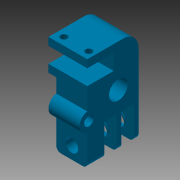
# Autodesk Inventor part: Part3
Saved by Autodesk Inventor 2015 (Build 190159000, 159)
## iProperties
Created: 2015-07-07
Part Number: Part3
Material: ABS Plastic
Document SubType Name: Modeling
Designer: eefred
Density: 1.06 g/cm^3
Appearance: Sky Blue Medium
Author: eefred
Autodesk Inventor part; units mm, degrees
ref_plane "YZ Plane" through (0, 0, 0) normal (1, 0, 0) x (0, 1, 0)
ref_plane "XZ Plane" through (0, 0, 0) normal (0, 1, 0) x (-1, 0, 0)
ref_plane "XY Plane" through (0, 0, 0) normal (0, 0, 1) x (1, 0, 0)
sketch "Sketch1" plane through (0, 0, 0) normal (1, 0, 0) x (0, 1, 0)
  line L0 (0, 0) -> (0, -5)
  line L1 (0, -5) -> (17, -5)
  line L2 (17, -5) -> (17, -15)
  line L3 (17, -15) -> (0, -15)
  line L4 (0, -61) -> (33, -61)
  line L5 (33, -61) -> (33, 0)
  line L6 (33, 0) -> (0, 0)
  circle A0 centre (1, -35) radius 3
  arc A1 (0, -29.0839) -> (0, -40.9161) centre (1, -35) ccw
  line L7 (0, -15) -> (0, -29.0839)
  line L8 (0, -61) -> (0, -40.9161)
  dimension "d0" = 5
  dimension "d1" = 17
  dimension "d2" = 10
  dimension "d4" = 33
  dimension "d6" = 6
  dimension "d7" = 1
  dimension "d8" = 20
  dimension "d9" = 6
  dimension "d47" = 46
  constraints: 18 end point, 5 perpendicular, 3 vertical, 2 centre point, 2 point on circle, 2 point on line, 1 coincident, 1 horizontal
  measures "d0" distance of L0.start L0.end
  measures "d1" distance of L0.end L1.end
  measures "d2" distance of L1.end L2.end
  measures "d4" distance of L4.start L4.end
  measures "d6" diameter of A0
  measures "d7" horizontal distance of L0.start A0.centre
  measures "d8" distance from line of L3 A0.centre
  measures "d9" radius of A1
  measures "d47" distance between parallel lines of L4 L3
extrude "Extrusion1" add sketch "Sketch1" along normal blind 25
sketch "Sketch2" plane through (0, 0, 0) normal (-1, 0, 0) x (0, 0, 1)
  line L0 (-70, -8) -> (-20, -8)
  line L1 (-20, -8) -> (-20, 42)
  line L2 (-20, 42) -> (-70, 42)
  line L3 (-70, 42) -> (-70, -8)
  point P0 (0, 0)
  dimension "d12" = 20
  dimension "d13" = 8
  dimension "d14" = 50
  dimension "d15" = 50
  constraints: 8 end point, 2 parallel, 1 horizontal, 1 perpendicular
  measures "d12" distance from line of point (0, 0) L1
  measures "d13" distance from line of point (0, 0) L0
  measures "d14" distance of L0.start L0.end
  measures "d15" distance of L2.end L0.start
extrude "Extrusion2" cut sketch "Sketch2" against normal blind 5
sketch "Sketch3" plane through (5, 0, 0) normal (-1, 0, 0) x (0, 0, 1)
  line L0 (-61, 22) -> (-40, 22)
  line L1 (-40, 22) -> (-40, 30)
  line L2 (-40, 30) -> (-61, 30)
  line L3 (-61, 30) -> (-61, 22)
  line L4 (-61, 11) -> (-40, 11)
  line L5 (-40, 11) -> (-40, 19)
  line L6 (-40, 19) -> (-61, 19)
  line L7 (-61, 19) -> (-61, 11)
  line L8 (-61, 33) -> (-20, 33) projected
  point P0 (0, 0)
  dimension "d18" = 8
  dimension "d19" = 8
  dimension "d20" = 21
  dimension "d21" = 3
  dimension "d22" = 3
  constraints: 16 end point, 4 parallel, 2 horizontal, 2 perpendicular, 2 point on line, 1 vertical alignment
  measures "d18" distance of L6.end L4.start
  measures "d19" distance of L2.end L0.start
  measures "d20" distance of L1.end L2.end
  measures "d21" distance between parallel lines of L0 L6
  measures "d22" distance between parallel lines of L8 L2
extrude "Extrusion3" cut sketch "Sketch3" against normal up to next
sketch "Sketch4" plane through (0, 33, 0) normal (0, 1, 0) x (1, 0, 0)
  circle A0 centre (15, 53) radius 4.1
  line L0 (5, 61) -> (25, 61) projected
  point P0 (0, 0)
  point P1 (15, 61)
  dimension "d25" = 8.2
  dimension "d26" = 8
  constraints: 1 centre point, 1 midpoint, 1 vertical alignment
  measures "d25" diameter of A0
  measures "d26" distance from line of L0 A0.centre
extrude "Extrusion4" cut sketch "Sketch4" against normal through all
sketch "Sketch5" plane through (5, 11, -40) normal (0, 1, 0) x (1, 0, 0)
  circle A0 centre (10, 13) radius 4.1 projected
  circle A1 centre (10, 13) radius 5
  point P0 (-5, -40)
  dimension "d29" = 10
  constraints: 1 centre point, 1 coincident
  measures "d29" diameter of A1
extrude "Extrusion5" add sketch "Sketch5" along normal blind 0.5
pattern_linear "Rectangular Pattern1" count 2 spacing 11 along (0, 1, 0) of "Extrusion5"
pattern_linear "Rectangular Pattern2" count 2 spacing 7.5 along (0, 1, 0) of "Extrusion5", "Rectangular Pattern1"
sketch "Sketch6" plane through (25, 0, 0) normal (1, 0, 0) x (0, 0, -1)
  circle A0 centre (27, 20) radius 6
  line L0 (61, 33) -> (0, 33) projected
  line L1 (0, 33) -> (0, 0) projected
  dimension "d38" = 12
  dimension "d39" = 13
  dimension "d40" = 27
  constraints: 1 centre point
  measures "d38" diameter of A0
  measures "d39" distance from line of L0 A0.centre
  measures "d40" distance from line of L1 A0.centre
extrude "Extrusion6" cut sketch "Sketch6" against normal up to surface (20 mm away)
fillet "Fillet1" radius 3 6 edges at (25, 31.5, -61) (25, 20.5, -61) (25, 5.5, -61) (5, 31.5, -61) (5, 20.5, -61) (5, 5.5, -61)
fillet "Fillet2" radius 10 1 edges at (12.5, 33, 0)
sketch "Sketch7" plane through (0, 33, -20) normal (0, 1, 0) x (1, 0, 0)
  spline S0 degree 2 poles (15.5392, -0.9329) (15.5392, -1.06) (15.5119, -1.3597) knots 0 0 0 1 1 1
  spline S1 degree 2 poles (15.5119, -1.3597) (15.4847, -1.6684) (15.4847, -1.8137) knots 0 0 0 1 1 1
  spline S2 degree 2 poles (15.4847, -1.8137) (15.4847, -3.2393) (15.9115, -4.5742) knots 0 0 0 1 1 1
  spline S3 degree 2 poles (15.9115, -4.5742) (16.084, -5.1281) (16.084, -5.3642) knots 0 0 0 1 1 1
  spline S4 degree 2 poles (16.084, -5.3642) (16.084, -5.682) (15.5846, -6.0362) (15.3576, -6.0362) knots 0 0 0 1 2 2 2
  spline S5 degree 2 poles (15.3576, -6.0362) (15.2577, -6.0362) (14.8763, -5.9454) knots 0 0 0 1 1 1
  spline S6 degree 2 poles (14.8763, -5.9454) (14.395, -5.8273) (13.7866, -5.7547) knots 0 0 0 1 1 1
  line L0 (13.7866, -5.7547) -> (9.4643, -5.2825)
  spline S7 degree 2 poles (9.4643, -5.2825) (8.8468, -5.228) (8.4836, -5.1372) (8.193, -4.774) (8.193, -4.4561) knots 0 0 0 1 2 3 3 3
  spline S8 degree 2 poles (8.193, -4.4561) (8.193, -4.211) (8.5653, -3.8296) (8.7832, -3.8296) knots 0 0 0 1 2 2 2
  spline S9 degree 2 poles (8.7832, -3.8296) (8.983, -3.8296) (9.4915, -3.9295) knots 0 0 0 1 1 1
  spline S10 degree 2 poles (9.4915, -3.9295) (10.227, -4.0657) (14.3678, -4.556) (14.4949, -4.556) knots 0 0 0 1 2 2 2
  spline S11 degree 2 poles (14.4949, -4.556) (14.6402, -4.556) (14.6402, -4.5015) knots 0 0 0 1 1 1
  spline S12 degree 2 poles (14.6402, -4.5015) (14.6402, -4.3018) (14.504, -3.4119) knots 0 0 0 1 1 1
  spline S13 degree 2 poles (14.504, -3.4119) (14.4313, -2.9942) (14.4132, -2.5674) knots 0 0 0 1 1 1
  spline S14 degree 2 poles (14.4132, -2.5674) (14.3587, -1.3506) (14.2316, -0.8602) knots 0 0 0 1 1 1
  spline S15 degree 2 poles (14.2316, -0.8602) (14.1952, -0.7059) (14.1952, -0.6332) knots 0 0 0 1 1 1
  spline S16 degree 2 poles (14.1952, -0.6332) (14.1952, -0.3426) (14.5403, -0.0157) (14.7764, -0.0157) knots 0 0 0 1 2 2 2
  spline S17 degree 2 poles (14.7764, -0.0157) (15.1215, -0.0157) (15.5392, -0.5787) (15.5392, -0.9329) knots 0 0 0 1 2 2 2
  point P0 (0, -20)
  point P1 (8.193, -6.6991)
  constraints: 1 other
extrude "Extrusion7" add sketch "Sketch7" along normal blind 0.5
sketch "Sketch8" plane through (0, 0, 0) normal (0, 0, 1) x (1, 0, 0)
  circle A0 centre (5, 5) radius 2.1
  circle A1 centre (21, 5) radius 2.1
  line L0 (0, 0) -> (25, 0) projected
  line L1 (25, 23) -> (25, 0) projected
  line L2 (0, 23) -> (0, 0) projected
  dimension "d48" = 4.2
  dimension "d49" = 5
  dimension "d50" = 4
  dimension "d51" = 5
  constraints: 2 centre point, 1 equal radius, 1 horizontal alignment
  measures "d48" diameter of A0
  measures "d49" distance from line of L0 A0.centre
  measures "d50" distance from line of L1 A1.centre
  measures "d51" distance from line of L2 A0.centre
extrude "Extrusion8" cut sketch "Sketch8" against normal up to next
equation "\"d18\" = d19"
equation "\"d21\" = d22"
body "Solid1"
